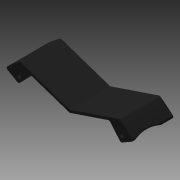
# Autodesk Inventor part: Bottom Plate Standoff
Saved by Autodesk Inventor 2015 (Build 190159000, 159)
## iProperties
Created: 2015-10-10
Part Number: Bottom Plate Standoff
Material: ABS Plastic
Document SubType Name: Modeling
Designer: James
Density: 1.06 g/cm^3
Appearance: Smooth - White
Mass: 185.582 g
Surface Area: 644.999 cm^2
Volume: 175.078 cm^3
Author: James
Autodesk Inventor part; units mm, degrees
ref_plane "YZ Plane" through (0, 0, 0) normal (1, 0, 0) x (0, 1, 0)
ref_plane "XZ Plane" through (0, 0, 0) normal (0, 1, 0) x (-1, 0, 0)
sketch "Sketch1" plane through (0, 0, 0) normal (0, 1, 0) x (-1, 0, 0)
  line L0 (-61.1122, 64.1506) -> (-69.0858, 68.7542)
  arc A0 (-69.4754, 71.9248) -> (-69.0858, 68.7542) centre (-68.0858, 70.4863) ccw
  arc A1 (-55.7942, 82.988) -> (-69.4754, 71.9248) centre (0, 0) ccw
  circle A2 centre (-56.8952, 69.5753) radius 3
  line L1 (-61.1122, 64.1506) -> (-58.2354, 62.4897)
  arc A3 (-69.4754, 71.9248) -> (-69.0858, 68.7542) centre (-68.0858, 70.4863) ccw
  arc A4 (-55.7942, 82.988) -> (-69.4754, 71.9248) centre (0, 0) ccw
  arc A5 (-58.2354, 62.4897) -> (-55.7033, 62.9362) centre (-57.2354, 64.2218) ccw
  line L2 (-69.0858, 68.7542) -> (-58.2354, 62.4897)
  arc A6 (-58.2354, 62.4897) -> (-55.7033, 62.9362) centre (-57.2354, 64.2218) ccw
  arc A7 (-69.4754, 71.9248) -> (-69.0858, 68.7542) centre (-68.0858, 70.4863) ccw
  arc A8 (-54.0401, 83.2237) -> (-55.7947, 82.9876) centre (-54.6783, 81.3283) ccw
  line L3 (-69.0858, 68.7542) -> (-58.2354, 62.4897)
  arc A9 (-54.0401, 83.2237) -> (-55.7947, 82.9876) centre (-54.6783, 81.3283) ccw
  arc A10 (-58.2354, 62.4897) -> (-55.7033, 62.9362) centre (-57.2354, 64.2218) ccw
  arc A11 (-69.4754, 71.9248) -> (-69.0858, 68.7542) centre (-68.0858, 70.4863) ccw
  arc A12 (-55.7947, 82.9876) -> (-69.4754, 71.9248) centre (0, 0) ccw
  arc A13 (-58.2354, 62.4897) -> (-55.7033, 62.9362) centre (-57.2354, 64.2218) ccw
  arc A14 (-69.4754, 71.9248) -> (-69.0858, 68.7542) centre (-68.0858, 70.4863) ccw
  arc A15 (-54.0401, 83.2237) -> (-55.7947, 82.9876) centre (-54.6783, 81.3283) ccw
  arc A16 (-55.7947, 82.9876) -> (-69.4754, 71.9248) centre (0, 0) ccw
  line L4 (-0.6382, 65.2434) -> (-54.0401, 83.2237)
  line L5 (61.1122, 64.1506) -> (69.0858, 68.7542)
  arc A17 (69.0858, 68.7542) -> (69.4754, 71.9248) centre (68.0858, 70.4863) ccw
  arc A18 (69.4754, 71.9248) -> (55.7942, 82.988) centre (0, 0) ccw
  circle A19 centre (56.8952, 69.5753) radius 3
  line L6 (61.1122, 64.1506) -> (58.2354, 62.4897)
  arc A20 (69.0858, 68.7542) -> (69.4754, 71.9248) centre (68.0858, 70.4863) ccw
  arc A21 (69.4754, 71.9248) -> (55.7942, 82.988) centre (0, 0) ccw
  arc A22 (55.7033, 62.9362) -> (58.2354, 62.4897) centre (57.2354, 64.2218) ccw
  line L7 (69.0858, 68.7542) -> (58.2354, 62.4897)
  arc A23 (55.7033, 62.9362) -> (58.2354, 62.4897) centre (57.2354, 64.2218) ccw
  arc A24 (69.0858, 68.7542) -> (69.4754, 71.9248) centre (68.0858, 70.4863) ccw
  arc A25 (55.7947, 82.9876) -> (54.0401, 83.2237) centre (54.6783, 81.3283) ccw
  line L8 (69.0858, 68.7542) -> (58.2354, 62.4897)
  arc A26 (55.7947, 82.9876) -> (54.0401, 83.2237) centre (54.6783, 81.3283) ccw
  arc A27 (55.7033, 62.9362) -> (58.2354, 62.4897) centre (57.2354, 64.2218) ccw
  arc A28 (69.0858, 68.7542) -> (69.4754, 71.9248) centre (68.0858, 70.4863) ccw
  arc A29 (69.4754, 71.9248) -> (55.7947, 82.9876) centre (0, 0) ccw
  arc A30 (55.7033, 62.9362) -> (58.2354, 62.4897) centre (57.2354, 64.2218) ccw
  arc A31 (69.0858, 68.7542) -> (69.4754, 71.9248) centre (68.0858, 70.4863) ccw
  arc A32 (55.7947, 82.9876) -> (54.0401, 83.2237) centre (54.6783, 81.3283) ccw
  arc A33 (69.4754, 71.9248) -> (55.7947, 82.9876) centre (0, 0) ccw
  line L9 (0.6382, 65.2434) -> (54.0401, 83.2237)
  line L10 (0.6382, 62.2149) -> (42.7519, 76.3945)
  line L11 (55.7033, 62.9362) -> (44.9222, 75.7846)
  arc A34 (44.9222, 75.7846) -> (42.7519, 76.3945) centre (43.3901, 74.499) ccw
  line L12 (-0.6382, 62.2149) -> (-42.7519, 76.3945)
  line L13 (-55.7033, 62.9362) -> (-44.9222, 75.7846)
  arc A35 (-42.7519, 76.3945) -> (-44.9222, 75.7846) centre (-43.3901, 74.499) ccw
  arc A36 (-0.6382, 65.2434) -> (0.6382, 65.2434) centre (0, 67.1389) ccw
  arc A37 (-0.6382, 62.2149) -> (0.6382, 62.2149) centre (0, 64.1103) ccw
  point P0 (-56.782, 61.6506)
  point P1 (0, 62)
  point P2 (0, 65.0285)
  point P3 (56.782, 61.6506)
  dimension "d36" = 2
  dimension "d59" = 2
  dimension "d60" = 2
  constraints: 74 point on circle, 38 centre point, 28 end point, 20 coincident, 8 tangent, 6 point on line, 2 collinear, 1 equal radius
  measures "d36" radius of A5
  measures "d59" radius of A34
  measures "d60" radius of A36
extrude "Extrusion1" add sketch "Sketch1" along normal blind 45
ref_plane "Work Plane2" through (93.3346, 0, 82.7542) normal (-0.8660254, 0, -0.5) x (0, 1, 0)
ref_plane "Work Plane1" through (69.0858, 0, 68.7542) normal (-0.8660254, 0, -0.5) x (0, 1, 0)
sketch "Sketch6" plane through (93.3346, 0, 82.7542) normal (-0.8660254, 0, -0.5) x (0, 1, 0)
  line L0 (17, 0) -> (32, 0)
  line L1 (17, 0) -> (2, 0)
  arc A0 (2, 0) -> (32, 0) centre (17, 36) ccw
  point P0 (0, 25)
  point P1 (0, 0)
  dimension "d44" = 17
  dimension "d45" = 15
  constraints: 4 end point, 2 point on circle, 1 centre point
  measures "d44" distance of point (0, 0) L0.start
  measures "d45" distance of L0.start L0.end
extrude "Extrusion7" cut sketch "Sketch6" along normal blind 85.903
mirror "Mirror3" about plane through (0, 0, 0) normal (1, 0, 0) of "Extrusion7"
fillet "Fillet1" radius 1 8 edges at (-69.1384, 17, 72.2487) (-70.029, 6.0744, 70.9597) (-70.029, 27.9256, 70.9597) (-63.6606, 2, 65.622) (-63.6606, 32, 65.622) (-56.4732, 4.029, 62.3727) (-56.4732, 29.971, 62.3727) (-54.8239, 17, 63.9842)
fillet "Fillet2" radius 1 8 edges at (69.1384, 17, 72.2487) (70.0297, 27.9349, 70.9569) (70.0297, 6.0651, 70.9569) (63.6606, 32, 65.622) (63.6606, 2, 65.622) (56.4712, 29.9664, 62.3735) (56.4712, 4.0336, 62.3735) (54.8239, 17, 63.9842)
body "Solid1"
